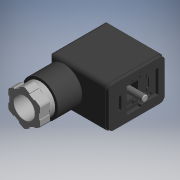
# Autodesk Inventor part: 34431 MSSD-F---(0)
Saved by Autodesk Inventor 2017.3 (Build 213256000, 256)
## iProperties
Part Number: 34431 MSSD-F---(0)
Material: Generic
Catalog Web Link: www.cadenas.de
Description: MSSD-Plug socket
Vendor: FESTO
Document SubType Name: Modeling
Designer: partserver
Manufacturer: FESTO
Mass: 17 g
Surface Area: 70.0007 cm^2
Volume: 20.4348 cm^3
Density: 1 g/cm^3
Appearance: PSOLRGB-79-79-79
Category: PARTsolutions
Company: FESTO
Title: 34431 MSSD-F
Author: Cadenas PARTsolutions
Comments: Plug socket
PSOL_IDENT_0: {$CADENAS_DATA\23d-libs\festo\parts\m\mssd\mssd.prj},175 {VTYP=3D},{NB=34431 MSSD-F---(0)},{LINA=344
PSOL_IDENT_1: 31 MSSD-F},{NN=MSSD},{DATE=11.01.2021 13:48:15},{GEOMDATE=11.01.2021 13:47:56},{VERSION=},{LINEID=15
PSOL_IDENT_2: 0},{WBVAR=POS},{WBNUMERIC=POS}  {NB=34431 MSSD-F---(0)},{LINA=34431 MSSD-F},{KT=DUMMY},{TNR=34431},{
PSOL_IDENT_3: TYP=MSSD-F},{INFO=},{VERS=15},{POS=0},{CNSMASSEXACT=0.017},{POSW=[0:180/180]},{EOLDATE=}
NB: 34431 MSSD-F---(0)
NN: MSSD
NT: Plug socket
NBSYN: $TNR. $TYP.---($POS.)
LINA: 34431 MSSD-F
CATALOG: Festo
TNR: 34431
TYP: MSSD-F
POS: 0
CNSMASSEXACT: 0.017
SUPPLIER: FESTO
ARTICLENO: 34431 MSSD-F---(0)
BOMINFO: 34431 MSSD-F
CREATOR: CADENAS GmbH
Autodesk Inventor part; units mm, degrees
ref_plane "YZ Plane" through (0, 0, 0) normal (1, 0, 0) x (0, 1, 0)
ref_plane "XZ Plane" through (0, 0, 0) normal (0, 1, 0) x (-1, 0, 0)
ref_plane "XY Plane" through (0, 0, 0) normal (0, 0, 1) x (1, 0, 0)
sketch "Skizze_1" plane through (0, 0, 0) normal (0, 0, 1) x (1, 0, 0)
  line L0 (-20.7, -14.3) -> (5.5, -14.3)
  arc A0 (5.5, -14.3) -> (7.5, -12.3) centre (5.5, -12.3) ccw
  line L1 (7.5, -12.3) -> (7.5, 12.3)
  arc A1 (7.5, 12.3) -> (5.5, 14.3) centre (5.5, 12.3) ccw
  line L2 (5.5, 14.3) -> (-20.7, 14.3)
  line L3 (-20.7, 14.3) -> (-20.7, -14.3)
  constraints: 8 end point, 4 point on circle, 2 centre point
extrude "Extrusion1" add sketch "Skizze_1" along normal mid plane 20.8
sketch "Skizze_3" plane through (0, 0, 0) normal (0, 1, 0) x (-1, 0, 0)
  arc A0 (-7.5, -8.4) -> (-5.5, -10.4) centre (-5.5, -8.4) ccw
  line L0 (-7.5, -8.4) -> (-7.5, 8.4)
  arc A1 (-5.5, 10.4) -> (-7.5, 8.4) centre (-5.5, 8.4) ccw
  line L1 (-5.5, 10.4) -> (-27.5, 10.4)
  line L2 (-27.5, 10.4) -> (-27.5, -10.4)
  line L3 (-27.5, -10.4) -> (-5.5, -10.4)
  constraints: 8 end point, 4 point on circle, 2 centre point
extrude "Extrusion2" cut sketch "Skizze_3" along normal mid plane 54
sketch "Skizze_2" plane through (-20.7, 0, 0) normal (1, 0, 0) x (0, 0, -1)
  line L0 (-16, -20) -> (16, -20)
  line L1 (16, -20) -> (16, 20)
  line L2 (16, 20) -> (-16, 20)
  line L3 (-16, 20) -> (-16, -20)
  arc A0 (-10.4, -12.3) -> (-8.4, -14.3) centre (-8.4, -12.3) ccw
  line L4 (-8.4, -14.3) -> (8.4, -14.3)
  arc A1 (8.4, -14.3) -> (10.4, -12.3) centre (8.4, -12.3) ccw
  line L5 (10.4, -12.3) -> (10.4, 12.3)
  arc A2 (10.4, 12.3) -> (8.4, 14.3) centre (8.4, 12.3) ccw
  line L6 (8.4, 14.3) -> (-8.4, 14.3)
  arc A3 (-8.4, 14.3) -> (-10.4, 12.3) centre (-8.4, 12.3) ccw
  line L7 (-10.4, 12.3) -> (-10.4, -12.3)
  constraints: 16 end point, 8 point on circle, 4 centre point
extrude "Extrusion3" cut sketch "Skizze_2" along normal blind 30
sketch "Skizze_6" plane through (-20.7, 0, 0) normal (1, 0, 0) x (0, 0, -1)
  arc A0 (-3.2, -3.1) -> (-3.1, -3.2) centre (-3.1, -3.1) ccw
  line L0 (-3.1, -3.2) -> (3.1, -3.2)
  arc A1 (3.1, -3.2) -> (3.2, -3.1) centre (3.1, -3.1) ccw
  line L1 (3.2, -3.1) -> (3.2, 3.1)
  arc A2 (3.2, 3.1) -> (3.1, 3.2) centre (3.1, 3.1) ccw
  line L2 (3.1, 3.2) -> (-3.1, 3.2)
  arc A3 (-3.1, 3.2) -> (-3.2, 3.1) centre (-3.1, 3.1) ccw
  line L3 (-3.2, 3.1) -> (-3.2, -3.1)
  constraints: 8 end point, 8 point on circle, 4 centre point
extrude "Extrusion4" cut sketch "Skizze_6" along normal blind 7.4
sketch "Sketch_5" plane through (-20.7, 0, 0) normal (1, 0, 0) x (0, 0, -1)
  arc A0 (-5.5, -4.05) -> (-5.3, -4.25) centre (-5.3, -4.05) ccw
  line L0 (-5.3, -4.25) -> (5.3, -4.25)
  arc A1 (5.3, -4.25) -> (5.5, -4.05) centre (5.3, -4.05) ccw
  line L1 (5.5, -4.05) -> (5.5, 0.05)
  arc A2 (5.5, 0.05) -> (5.3, 0.25) centre (5.3, 0.05) ccw
  line L2 (5.3, 0.25) -> (4.1, 0.25)
  line L3 (4.1, 0.25) -> (4.1, 7.05)
  arc A3 (4.1, 7.05) -> (3.9, 7.25) centre (3.9, 7.05) ccw
  line L4 (3.9, 7.25) -> (2.25, 7.25)
  line L5 (2.25, 7.25) -> (2.25, 8.05)
  arc A4 (2.25, 8.05) -> (2.05, 8.25) centre (2.05, 8.05) ccw
  line L6 (2.05, 8.25) -> (-2.05, 8.25)
  arc A5 (-2.05, 8.25) -> (-2.25, 8.05) centre (-2.05, 8.05) ccw
  line L7 (-2.25, 8.05) -> (-2.25, 7.25)
  line L8 (-2.25, 7.25) -> (-3.9, 7.25)
  arc A6 (-3.9, 7.25) -> (-4.1, 7.05) centre (-3.9, 7.05) ccw
  line L9 (-4.1, 7.05) -> (-4.1, 0.25)
  line L10 (-4.1, 0.25) -> (-5.3, 0.25)
  arc A7 (-5.3, 0.25) -> (-5.5, 0.05) centre (-5.3, 0.05) ccw
  line L11 (-5.5, 0.05) -> (-5.5, -4.05)
  constraints: 24 end point, 16 point on circle, 8 centre point
extrude "Extrusion5" cut sketch "Sketch_5" along normal blind 1
sketch "Sketch_6" plane through (-20.7, 0, 0) normal (1, 0, 0) x (0, 0, -1)
  line L0 (-8.9, 12.8) -> (-8.9, -12.8)
  line L1 (-8.9, -12.8) -> (8.9, -12.8)
  line L2 (8.9, -12.8) -> (8.9, 12.8)
  line L3 (8.9, 12.8) -> (-8.9, 12.8)
  constraints: 8 end point
extrude "Extrusion6" cut sketch "Sketch_6" along normal blind 0.5
sketch "Skizze_5" plane through (0, 0, 0) normal (0, 0, 1) x (1, 0, 0)
  line L0 (0, -34.5) -> (0, -9.6015)
  line L1 (0, -9.6015) -> (7.2899, -9.6015)
  line L2 (7.2899, -9.6015) -> (9, -14.3)
  line L3 (9, -14.3) -> (9, -26.3)
  arc A0 (8.8, -26.5) -> (9, -26.3) centre (8.8, -26.3) ccw
  line L4 (8.8, -26.5) -> (7.6, -26.5)
  line L5 (7.6, -26.5) -> (7.6, -29.5)
  line L6 (7.6, -29.5) -> (9, -29.5)
  line L7 (9, -29.5) -> (9, -34.5)
  line L8 (9, -34.5) -> (5.45, -34.5)
  arc A1 (5.25, -34.3) -> (5.45, -34.5) centre (5.45, -34.3) ccw
  line L9 (5.25, -34.3) -> (5.25, -26.5)
  line L10 (5.25, -26.5) -> (0, -26.5)
  line L11 (0, -26.5) -> (0, -9.6015)
  constraints: 24 end point, 4 point on circle, 2 centre point
revolve "Revolution1" add sketch "Skizze_5" angle 360 about axis through (0, -34.5, 0) along (0, -1, 0)
sketch "Skizze_15" plane through (0, -34.5, 0) normal (0, 1, 0) x (1, 0, 0)
  line L0 (-14, -14) -> (14, -14)
  line L1 (14, -14) -> (14, 14)
  line L2 (14, 14) -> (-14, 14)
  line L3 (-14, 14) -> (-14, -14)
  line L4 (-8, -1.5) -> (-8, -4.6188)
  line L5 (-8, -4.6188) -> (-5.299, -6.1782)
  line L6 (-5.299, -6.1782) -> (-5.049, -5.7452)
  line L7 (-5.049, -5.7452) -> (-2.451, -7.2452)
  line L8 (-2.451, -7.2452) -> (-2.701, -7.6782)
  line L9 (-2.701, -7.6782) -> (0, -9.2376)
  line L10 (0, -9.2376) -> (2.701, -7.6782)
  line L11 (2.701, -7.6782) -> (2.451, -7.2452)
  line L12 (2.451, -7.2452) -> (5.049, -5.7452)
  line L13 (5.049, -5.7452) -> (5.299, -6.1782)
  line L14 (5.299, -6.1782) -> (8, -4.6188)
  line L15 (8, -4.6188) -> (8, -1.5)
  line L16 (8, -1.5) -> (7.5, -1.5)
  line L17 (7.5, -1.5) -> (7.5, 1.5)
  line L18 (7.5, 1.5) -> (8, 1.5)
  line L19 (8, 1.5) -> (8, 4.6188)
  line L20 (8, 4.6188) -> (5.299, 6.1782)
  line L21 (5.299, 6.1782) -> (5.049, 5.7452)
  line L22 (5.049, 5.7452) -> (2.451, 7.2452)
  line L23 (2.451, 7.2452) -> (2.701, 7.6782)
  line L24 (2.701, 7.6782) -> (0, 9.2376)
  line L25 (0, 9.2376) -> (-2.701, 7.6782)
  line L26 (-2.701, 7.6782) -> (-2.451, 7.2452)
  line L27 (-2.451, 7.2452) -> (-5.049, 5.7452)
  line L28 (-5.049, 5.7452) -> (-5.299, 6.1782)
  line L29 (-5.299, 6.1782) -> (-8, 4.6188)
  line L30 (-8, 4.6188) -> (-8, 1.5)
  line L31 (-8, 1.5) -> (-7.5, 1.5)
  line L32 (-7.5, 1.5) -> (-7.5, -1.5)
  line L33 (-7.5, -1.5) -> (-8, -1.5)
  constraints: 68 end point
extrude "Extrusion7" cut sketch "Skizze_15" along normal blind 5
sketch "Skizze_8" plane through (-20.7, 0, 0) normal (1, 0, 0) x (0, 0, -1)
  line L0 (4.95, 2.65) -> (6.05, 2.65)
  line L1 (6.05, 2.65) -> (6.05, 9.35)
  line L2 (6.05, 9.35) -> (4.95, 9.35)
  line L3 (4.95, 9.35) -> (4.95, 2.65)
  constraints: 8 end point
extrude "Extrusion8" cut sketch "Skizze_8" along normal blind 12
sketch "Skizze_9" plane through (-20.7, 0, 0) normal (1, 0, 0) x (0, 0, -1)
  line L0 (-6.05, 2.65) -> (-4.95, 2.65)
  line L1 (-4.95, 2.65) -> (-4.95, 9.35)
  line L2 (-4.95, 9.35) -> (-6.05, 9.35)
  line L3 (-6.05, 9.35) -> (-6.05, 2.65)
  constraints: 8 end point
extrude "Extrusion9" cut sketch "Skizze_9" along normal blind 12
sketch "Skizze_10" plane through (-20.7, 0, 0) normal (1, 0, 0) x (0, 0, -1)
  line L0 (-3.35, -9.05) -> (3.35, -9.05)
  line L1 (3.35, -9.05) -> (3.35, -7.95)
  line L2 (3.35, -7.95) -> (-3.35, -7.95)
  line L3 (-3.35, -7.95) -> (-3.35, -9.05)
  constraints: 8 end point
extrude "Extrusion10" cut sketch "Skizze_10" along normal blind 12
sketch "Skizze_11" plane through (0, 0, 0) normal (0, 0, 1) x (1, 0, 0)
  line L0 (8, 0) -> (5, 0)
  line L1 (5, 0) -> (5, 3)
  line L2 (5, 3) -> (8, 3)
  line L3 (8, 3) -> (8, 0)
  line L4 (8, 0) -> (5, 0)
  constraints: 10 end point
revolve "Revolution2" cut sketch "Skizze_11" angle 360 about axis through (8, 0, 0) along (1, 0, 0)
sketch "Skizze_12" plane through (0, 0, 0) normal (0, 0, 1) x (1, 0, 0)
  line L0 (7, 0) -> (-26.5, 0)
  line L1 (-26.5, 0) -> (-26.5, 1.1935)
  line L2 (-26.5, 1.1935) -> (-26.1935, 1.5)
  line L3 (-26.1935, 1.5) -> (5, 1.5)
  line L4 (5, 1.5) -> (5, 2.75)
  line L5 (5, 2.75) -> (7, 2.75)
  line L6 (7, 2.75) -> (7, 0)
  line L7 (7, 0) -> (-26.5, 0)
  constraints: 16 end point
revolve "Revolution3" add sketch "Skizze_12" angle 360 about axis through (7, 0, 0) along (1, 0, 0)
thread "Thread1" size "M3x0.5" class "6g" standard "ISO Metric profile" length 31.1935
sketch "Skizze_13" plane through (7, 0, 0) normal (1, 0, 0) x (0, 0, -1)
  arc A0 (-2.7208, 0.4) -> (-2.7208, -0.4) centre (0, 0) ccw
  line L0 (-2.7208, -0.4) -> (-0.4, -0.4)
  line L1 (-0.4, -0.4) -> (-0.4, -2.7208)
  arc A1 (-0.4, -2.7208) -> (0.4, -2.7208) centre (0, 0) ccw
  line L2 (0.4, -2.7208) -> (0.4, -0.4)
  line L3 (0.4, -0.4) -> (2.7208, -0.4)
  arc A2 (2.7208, -0.4) -> (2.7208, 0.4) centre (0, 0) ccw
  line L4 (2.7208, 0.4) -> (0.4, 0.4)
  line L5 (0.4, 0.4) -> (0.4, 2.7208)
  arc A3 (0.4, 2.7208) -> (-0.4, 2.7208) centre (0, 0) ccw
  line L6 (-0.4, 2.7208) -> (-0.4, 0.4)
  line L7 (-0.4, 0.4) -> (-2.7208, 0.4)
  constraints: 16 end point, 8 point on circle, 4 centre point
extrude "Extrusion11" cut sketch "Skizze_13" against normal blind 1.2
sketch "Sketch_7" plane through (-20.7, 0, 0) normal (1, 0, 0) x (0, 0, -1)
  arc A0 (-10.1, -11.65) -> (-7.6, -14.15) centre (-7.6, -11.65) ccw
  line L0 (-7.6, -14.15) -> (7.6, -14.15)
  arc A1 (7.6, -14.15) -> (10.1, -11.65) centre (7.6, -11.65) ccw
  line L1 (10.1, -11.65) -> (10.1, 11.65)
  arc A2 (10.1, 11.65) -> (7.6, 14.15) centre (7.6, 11.65) ccw
  line L2 (7.6, 14.15) -> (-7.6, 14.15)
  arc A3 (-7.6, 14.15) -> (-10.1, 11.65) centre (-7.6, 11.65) ccw
  line L3 (-10.1, 11.65) -> (-10.1, -11.65)
  arc A4 (-2.8, -7.8) -> (-2.8, -8.9) centre (-2.8, -8.35) ccw
  line L4 (-2.8, -8.9) -> (2.8, -8.9)
  arc A5 (2.8, -8.9) -> (2.8, -7.8) centre (2.8, -8.35) ccw
  line L5 (2.8, -7.8) -> (-2.8, -7.8)
  arc A6 (-6.9, -4.95) -> (-6.7, -5.15) centre (-6.7, -4.95) ccw
  line L6 (-6.7, -5.15) -> (6.7, -5.15)
  arc A7 (6.7, -5.15) -> (6.9, -4.95) centre (6.7, -4.95) ccw
  line L7 (6.9, -4.95) -> (6.9, 1.95)
  arc A8 (6.9, 1.95) -> (6.7, 2.15) centre (6.7, 1.95) ccw
  line L8 (6.7, 2.15) -> (6.1, 2.15)
  arc A9 (5.9, 2.35) -> (6.1, 2.15) centre (6.1, 2.35) ccw
  line L9 (5.9, 2.35) -> (5.9, 10.75)
  arc A10 (5.9, 10.75) -> (5.7, 10.95) centre (5.7, 10.75) ccw
  line L10 (5.7, 10.95) -> (-5.7, 10.95)
  arc A11 (-5.7, 10.95) -> (-5.9, 10.75) centre (-5.7, 10.75) ccw
  line L11 (-5.9, 10.75) -> (-5.9, 2.35)
  arc A12 (-6.1, 2.15) -> (-5.9, 2.35) centre (-6.1, 2.35) ccw
  line L12 (-6.1, 2.15) -> (-6.7, 2.15)
  arc A13 (-6.7, 2.15) -> (-6.9, 1.95) centre (-6.7, 1.95) ccw
  line L13 (-6.9, 1.95) -> (-6.9, -4.95)
  constraints: 28 end point, 28 point on circle, 14 centre point
extrude "Extrusion12" add sketch "Sketch_7" against normal blind 1.5
ref_plane "2SOC_XY" through (-22.2, 0, 0) normal (1, 0, 0) x (0, 0, -1)
ref_plane "2SOC_YZ" through (-22.2, 0, 0) normal (0, 0, -1) x (0, 1, 0)
ref_plane "2SOC_ZX" through (-22.2, 0, 0) normal (0, 1, 0) x (1, 0, 0)
ref_plane "ANBAU_XY" through (-22.2, 0, 0) normal (1, 0, 0) x (0, 0, -1)
ref_plane "ANBAU_YZ" through (-22.2, 0, 0) normal (0, 0, -1) x (0, 1, 0)
ref_plane "ANBAU_ZX" through (-22.2, 0, 0) normal (0, 1, 0) x (1, 0, 0)
body "Solid1"
